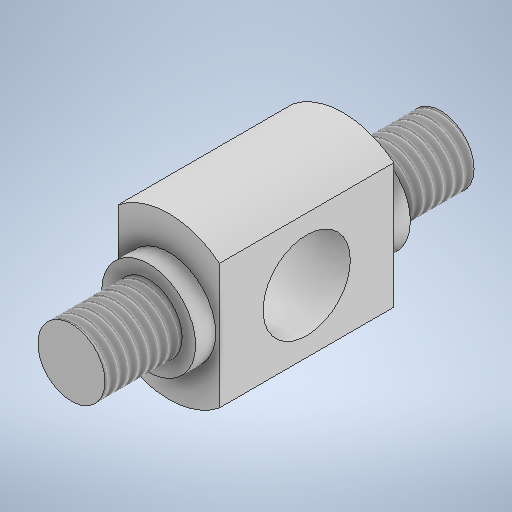
# Autodesk Inventor part: Pieza 11
Saved by Autodesk Inventor 2025.3 (Build 293356030, 356C)
## iProperties
Created: 2025-08-24
Part Number: Pieza 11
Material: Generic
Document SubType Name: Modeling
Designer: PC
Density: 1 g/cm^3
Appearance: Default
Author: PC
Autodesk Inventor part; units mm, degrees
ref_plane "YZ Plane" through (0, 0, 0) normal (1, 0, 0) x (0, 1, 0)
ref_plane "XZ Plane" through (0, 0, 0) normal (0, 1, 0) x (-1, 0, 0)
sketch "Sketch1" plane through (0, 0, 0) normal (0, 0, 1) x (1, 0, 0)
  line L0 (7.5517, 9.3259) -> (7.5517, -9.3259)
  line L1 (-7.5517, -9.3259) -> (-7.5517, 9.3259)
  line L2 (-7.5517, 9.3259) -> (7.5517, -9.3259) construction
  line L3 (7.5517, 9.3259) -> (-7.5517, -9.3259) construction
  arc A0 (-7.5517, -9.3259) -> (7.5517, -9.3259) centre (0, 0) ccw
  arc A1 (7.5517, 9.3259) -> (-7.5517, 9.3259) centre (0, 0) ccw
  constraints: 8 end point, 4 point on circle, 2 centre point, 2 midpoint, 1 coincident, 1 parallel
extrude "Extrusion1" add sketch "Sketch1" along normal blind 26
sketch "Sketch2" plane through (0, 0, 26) normal (0, 0, 1) x (1, 0, 0)
  circle A0 centre (0, 0) radius 7
  dimension "d3" = 14
  constraints: 1 centre point, 1 coincident
  measures "d3" diameter of A0
extrude "Extrusion2" add sketch "Sketch2" along normal blind 3
sketch "Sketch3" plane through (0, 0, 29) normal (0, 0, 1) x (1, 0, 0)
  circle A0 centre (0, 0) radius 5
  dimension "d6" = 10
  constraints: 1 centre point, 1 coincident
  measures "d6" diameter of A0
extrude "Extrusion3" add sketch "Sketch3" along normal blind 11.5
ref_plane "Work Plane1" through (0, 0, 13) normal (0, 0, 1) x (1, 0, 0)
mirror "Mirror1" about plane through (0, 0, 13) normal (0, 0, 1) of "Extrusion3", "Extrusion2"
sketch "Sketch4" plane through (-7.5517, -9.3259, 0) normal (-1, 0, 0) x (0, 0, 1)
  circle A0 centre (13, 9.3259) radius 6.5
  point P0 (0, 9.3259)
  dimension "d9" = 13
  constraints: 1 centre point, 1 coincident
  measures "d9" diameter of A0
extrude "Extrusion4" cut sketch "Sketch4" against normal blind 100
thread "Thread1" size "M10x1.5" class "6g" standard "ANSI Metric M Profile" length 13
thread "Thread2" size "M10x1.5" class "6g" standard "ISO Metric profile" length 13
body "Solid1"
